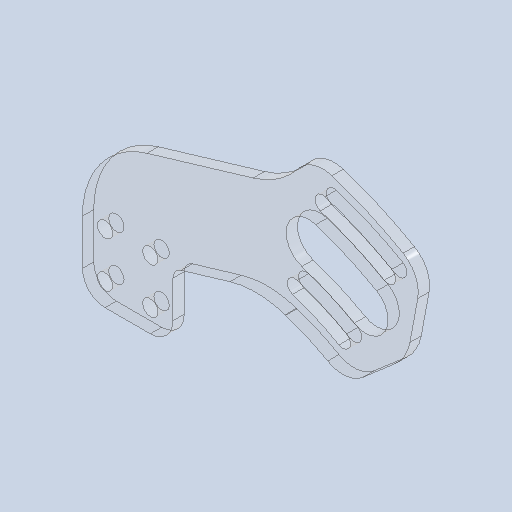
# Autodesk Inventor part: IntakeForearm
Saved by Autodesk Inventor 2023 (Build 270158000, 158)
## iProperties
Created: 2022-11-09
Part Number: IntakeForearm
Material: Polycarbonate, Clear
Document SubType Name: Modeling
Designer: Zac Hah
Density: 1.2 g/cm^3
Appearance: Polycarbonate - Clear
Author: Zac Hah
Autodesk Inventor part; units mm, degrees
ref_plane "YZ Plane" through (0, 0, 0) normal (1, 0, 0) x (0, 1, 0)
ref_plane "XZ Plane" through (0, 0, 0) normal (0, 1, 0) x (-1, 0, 0)
ref_plane "XY Plane" through (0, 0, 0) normal (0, 0, 1) x (1, 0, 0)
sketch "Sketch1" plane through (0, 0, 0) normal (0, 0, 1) x (1, 0, 0)
  arc A0 (-0.0635, 21.727) -> (-1.9234, 26.2171) centre (-6.4135, 21.727) ccw projected
  line L0 (-12.7635, 37.0572) -> (-1.9234, 26.2171) projected
  arc A1 (-12.7635, 37.0572) -> (-22.9837, 35.3037) centre (-17.2536, 32.5671) ccw projected
  arc A2 (-22.9837, 35.3037) -> (-25.4635, 24.3572) centre (-0.0635, 24.3572) ccw projected
  line L1 (-25.4635, 8.4822) -> (-25.4635, 24.3572) projected
  arc A3 (-25.4635, 8.4822) -> (-20.3429, -6.8118) centre (-0.0635, 8.4822) ccw projected
  line L2 (2.6238, -37.2648) -> (-20.3429, -6.8118) projected
  arc A4 (2.6238, -37.2648) -> (22.9032, -21.9707) centre (12.7635, -29.6178) ccw projected
  line L3 (1.2167, 6.7848) -> (22.9032, -21.9707) projected
  arc A5 (-0.0635, 10.6083) -> (1.2167, 6.7848) centre (6.2865, 10.6083) ccw projected
  line L4 (-0.0635, 21.727) -> (-0.0635, 10.6083) projected
  circle A6 centre (-19.1135, 24.3572) radius 2.159 projected
  circle A7 centre (-6.4135, 24.3572) radius 2.159 projected
  circle A8 centre (-6.4135, -13.7428) radius 2.159 projected
  circle A9 centre (-6.4135, -1.0428) radius 2.159 projected
  circle A10 centre (-6.4135, 11.6572) radius 2.159 projected
  circle A11 centre (-19.1135, 11.6572) radius 2.159 projected
  circle A12 centre (12.7635, -29.6178) radius 2.159 projected
  line L5 (81.8636, -46.7367) -> (81.8636, 125.7735) construction
  line L6 (61.5605, 6.4848) -> (81.5605, 6.4848) construction
  line L7 (81.5605, 6.4848) -> (81.5605, 146.4848) construction
  line L8 (81.5605, 146.4848) -> (61.5605, 146.4848) construction
  line L9 (61.5605, 146.4848) -> (61.5605, 6.4848) construction
  circle A13 centre (53.9115, 41.9458) radius 25.4 construction
  arc A14 (49.9598, 13.7707) -> (6.7541, 27.2154) centre (12.7635, -29.6178) ccw construction
  arc A15 (53.9115, 41.9458) -> (38.0365, 48.9684) centre (12.7635, -29.6178) ccw construction
  arc A16 (57.0767, 47.4507) -> (39.9806, 55.0134) centre (12.7635, -29.6178) ccw
  arc A17 (50.7463, 36.4409) -> (36.0924, 42.9233) centre (12.7635, -29.6178) ccw
  arc A18 (50.7463, 36.4409) -> (57.0767, 47.4507) centre (53.9115, 41.9458) ccw
  arc A19 (39.9806, 55.0134) -> (36.0924, 42.9233) centre (38.0365, 48.9684) ccw
  circle A20 centre (38.0365, 48.9684) radius 25.4 construction
  arc A21 (53.9115, 41.9458) -> (38.0365, 48.9684) centre (12.7635, -29.6178) ccw construction
  arc A22 (60.242, 52.9556) -> (41.9247, 61.0585) centre (12.7635, -29.6178) ccw construction
  arc A23 (47.581, 30.936) -> (34.1483, 36.8782) centre (12.7635, -29.6178) ccw construction
  arc A24 (47.581, 30.936) -> (60.242, 52.9556) centre (53.9115, 41.9458) ccw
  arc A25 (41.9247, 61.0585) -> (34.1483, 36.8782) centre (38.0365, 48.9684) ccw construction
  circle A26 centre (-19.1135, 11.6572) radius 6.35
  circle A27 centre (-6.4135, 11.6572) radius 6.35
  line L10 (-6.4135, 5.3072) -> (-19.1135, 5.3072)
  line L11 (-0.0635, 21.727) -> (-0.0635, 24.3572)
  arc A28 (47.581, 30.936) -> (34.1483, 36.8782) centre (12.7635, -29.6178) ccw construction
  arc A29 (48.6572, 32.8077) -> (34.8093, 38.9335) centre (12.7635, -29.6178) ccw
  arc A30 (46.5049, 29.0644) -> (33.4874, 34.8229) centre (12.7635, -29.6178) ccw
  arc A31 (46.5049, 29.0644) -> (48.6572, 32.8077) centre (47.581, 30.936) ccw
  arc A32 (34.8093, 38.9335) -> (33.4874, 34.8229) centre (34.1483, 36.8782) ccw
  line L12 (38.0365, 48.9684) -> (12.7635, -29.6178) construction
  line L13 (53.9115, 41.9458) -> (12.7635, -29.6178) construction
  arc A33 (60.242, 52.9556) -> (41.9247, 61.0585) centre (12.7635, -29.6178) ccw construction
  arc A34 (61.3181, 54.8273) -> (42.5856, 63.1139) centre (12.7635, -29.6178) ccw
  arc A35 (59.1658, 51.0839) -> (41.2637, 59.0032) centre (12.7635, -29.6178) ccw
  arc A36 (59.1658, 51.0839) -> (61.3181, 54.8273) centre (60.242, 52.9556) ccw
  arc A37 (42.5856, 63.1139) -> (41.2637, 59.0032) centre (41.9247, 61.0585) ccw
  line L14 (38.0365, 48.9684) -> (41.9247, 61.0585) construction
  arc A38 (56.0006, 45.579) -> (39.3196, 52.9581) centre (12.7635, -29.6178) ccw
  arc A39 (56.0006, 45.579) -> (64.4834, 60.3321) centre (60.242, 52.9556) ccw
  arc A40 (64.4834, 60.3321) -> (44.5297, 69.1589) centre (12.7635, -29.6178) ccw
  arc A41 (44.5297, 69.1589) -> (39.3196, 52.9581) centre (41.9247, 61.0585) ccw
  arc A42 (51.8224, 38.3126) -> (36.7534, 44.9786) centre (12.7635, -29.6178) ccw
  arc A43 (36.7534, 44.9786) -> (31.5433, 28.7778) centre (34.1483, 36.8782) ccw
  arc A44 (43.3396, 23.5595) -> (31.5433, 28.7778) centre (12.7635, -29.6178) ccw
  arc A45 (43.3396, 23.5595) -> (51.8224, 38.3126) centre (47.581, 30.936) ccw
  line L15 (62.2155, 32.3368) -> (53.1447, 24.498)
  line L16 (66.3936, 39.6032) -> (68.605, 51.386)
  line L17 (34.4081, 61.139) -> (-7.3204, 48.6985)
  arc A46 (-7.3204, 48.6985) -> (-22.9837, 35.3037) centre (-0.0635, 24.3572) ccw
  line L18 (-0.0635, 24.3572) -> (37.7202, 35.6217)
  point P0 (0, 0)
  point P1 (-0.0635, 11.6572)
  point P2 (-25.4635, 11.6572)
  point P3 (-12.7635, 11.6572)
  point P4 (33.4184, 60.8439)
  point P5 (26.9132, 32.3998)
  dimension "d0" = 20
  dimension "d1" = 140
  dimension "d2" = 50.8
  dimension "d3" = 57.15
  dimension "d4" = 53.975
  dimension "d6" = 12.7
  dimension "d7" = 38.1
  dimension "d8" = 25.4
  dimension "d11" = 4.318
  dimension "d12" = 12.7
  dimension "d13" = 12.7
  dimension "d14" = 6.35
  dimension "d15" = 6.35
  constraints: 67 point on circle, 32 centre point, 28 end point, 24 tangent, 10 coincident, 4 vertical, 3 equal radius, 3 horizontal, 3 parallel, 3 point on line, 1 collinear, 1 perpendicular, 12 other
  measures "d0" distance of L8.end L7.end
  measures "d1" distance of L7.end L6.end
  measures "d2" diameter of A13
  measures "d3" radius of A14
  measures "d4" distance from line of L4 A13.centre
  measures "d6" diameter of A19
  measures "d7" distance from line of A15.end L4
  measures "d8" diameter of A25
  measures "d11" diameter of A32
  measures "d12" radial gap between concentric circles of A15 A28
  measures "d13" radial gap between concentric circles of A33 A21
  measures "d14" radial gap between concentric circles of A37 A41
  measures "d15" radial gap between concentric circles of A31 A45
extrude "Extrusion1" add sketch "Sketch1" along normal blind 3.175 contours L4 A27 A26 L1 A2 A1 L0 A0 | A0 L0 A1 A46 L17 A41 A19 A43 L18 L11 | A27 | A27 L10 A26 | A26 | L18 A30 A31 A24 A45 A44 A43 | A43 A19 A17 A18 A45 A24 A31 A29 A32 A30 L18 | A41 A40 A39 A18 A16 A19 | A45 A24 L15 | A18 A39 A24 A45 | A24 A39 L16
fillet "Fillet1" radius 25.4 2 edges at (26.9132, 32.3998, 1.5875) (33.4184, 60.8439, 1.5875)
fillet "Fillet2" radius 3.175 1 edges at (-0.0635, 24.3572, 1.5875)
body "Solid1"
